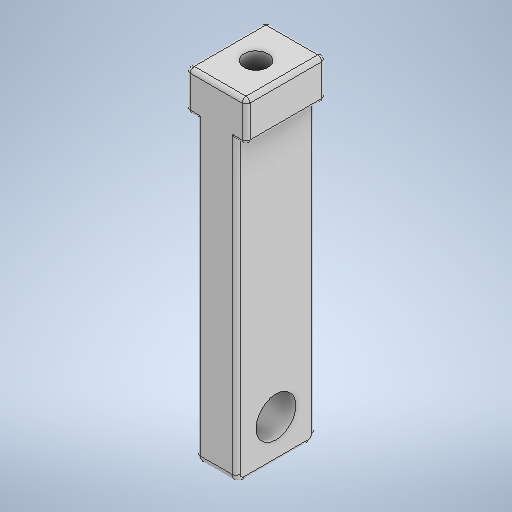
# Autodesk Inventor part: Suporte da base movel
Saved by Autodesk Inventor 2025.3 (Build 293356000, 356)
## iProperties
Created: 2025-02-14
Part Number: Suporte da base movel
Material: Generic
Document SubType Name: Modeling
Designer: erikg
Density: 1 g/cm^3
Appearance: Default
Author: erikg
Autodesk Inventor part; units mm, degrees
ref_plane "YZ Plane" through (0, 0, 0) normal (1, 0, 0) x (0, 1, 0)
ref_plane "XZ Plane" through (0, 0, 0) normal (0, 1, 0) x (-1, 0, 0)
ref_plane "XY Plane" through (0, 0, 0) normal (0, 0, 1) x (1, 0, 0)
sketch "Sketch1" plane through (0, 0, 0) normal (0, 0, 1) x (1, 0, 0)
  line L0 (0, 0) -> (10, 0)
  line L1 (10, 0) -> (10, 85)
  line L2 (10, 85) -> (0, 85)
  line L3 (0, 85) -> (0, 0)
  dimension "d0" = 10
  dimension "d1" = 85
  constraints: 8 end point, 2 parallel, 1 horizontal, 1 perpendicular
  measures "d0" distance of L1.end L2.end
  measures "d1" distance of L0.end L1.end
extrude "Extrusion1" add sketch "Sketch1" along normal mid plane 20
sketch "Sketch2" plane through (0, 0, 10) normal (-1, 0, 0) x (0, 0, 1)
  line L0 (-20, 0) -> (-20, 85) projected
  line L1 (-20, 0) -> (0, 0) projected
  line L2 (0, 85) -> (0, 0) projected
  point P0 (-10, 0)
  point P1 (-10, 10)
  point P2 (-10, 0)
  dimension "d14" = 10
  dimension "d15" = 10
  constraints: 1 midpoint
  measures "d14" distance from line of L0 point (-10, 10)
  measures "d15" distance from line of point (-10, 10) L1
hole "Hole1" at (0, 10, 0) direction (1, 0, 0) diameter 10 end through all
fillet "Fillet1" radius 2 2 edges at (5, 0, -10) (5, 0, 10)
sketch "Sketch4" plane through (0, 0, 0) normal (0, 0, 1) x (1, 0, 0)
  line L0 (-2.5, 85) -> (12.5, 85)
  line L1 (12.5, 85) -> (12.5, 75)
  line L2 (12.5, 75) -> (-2.5, 75)
  line L3 (-2.5, 75) -> (-2.5, 85)
  line L4 (10, 85) -> (0, 85) projected
  point P0 (0, 0)
  point P1 (5, 85)
  point P2 (5, 85)
  dimension "d27" = 15
  dimension "d28" = 10
  dimension "d29" = 7.5
  dimension "d32" = 0
  constraints: 8 end point, 2 midpoint, 2 parallel, 1 horizontal, 1 perpendicular
  measures "d27" distance of L1.end L2.end
  measures "d28" distance of L0.end L1.end
  measures "d29" distance from line of point (5, 85) L1
  measures "d32" distance from line of point (5, 85) L0
extrude "Extrusion3" add sketch "Sketch4" along normal mid plane 20
sketch "Sketch3" plane through (0, 85, 10) normal (0, 1, 0) x (1, 0, 0)
  circle A0 centre (5, 10) radius 3
  point P0 (0, 10)
  dimension "d24" = 6
  constraints: 1 centre point
  measures "d24" diameter of A0
extrude "Extrusion2" cut sketch "Sketch3" along normal blind 20 and the other way blind 18
fillet "Fillet2" radius 1 2 edges at (-2.5, 75, 0) (12.5, 75, 0)
fillet "Fillet3" radius 1 22 edges at (10, 0.5858, 9.4142) (10, 0, 0) (10, 0.5858, -9.4142) (10, 38.5, -10) (10, 38.5, 10) (0, 0.5858, 9.4142) (0, 0, 0) (0, 0.5858, -9.4142) (0, 38.5, -10) (0, 38.5, 10) (-0.75, 75, 10) (-2.5, 80.5, 10) (12.5, 85, 0) (-2.5, 85, 0) (5, 85, 10) (5, 85, -10) (10.75, 75, -10) (12.5, 80.5, -10) (10.75, 75, 10) (12.5, 80.5, 10) (-0.75, 75, -10) (-2.5, 80.5, -10)
equation "\"d15\" = d14"
equation "\"d29\" = 0.5 * d27"
body "Solid1"
